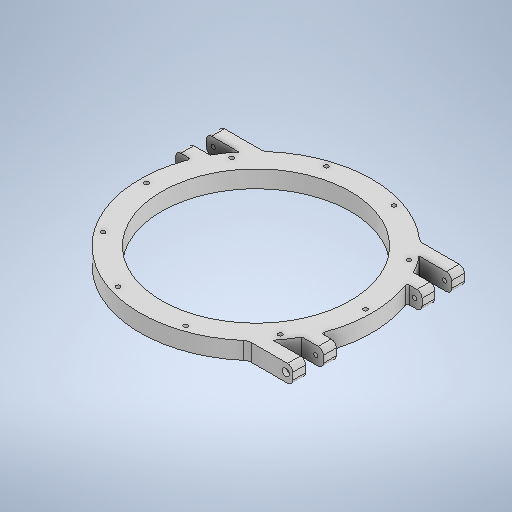
# Autodesk Inventor part: Cylinder 80-20 Spacer_2
Saved by Autodesk Inventor 2025 (Build 290162000, 162)
## iProperties
Created: 2024-04-28
Part Number: Cylinder 80-20 Spacer_2
Material: Generic
Document SubType Name: Modeling
Designer: Thienan Hoang
Density: 1 g/cm^3
Appearance: Default
Author: Thienan Hoang
Autodesk Inventor part; units mm, degrees
ref_plane "YZ Plane" through (0, 0, 0) normal (1, 0, 0) x (0, 1, 0)
ref_plane "XZ Plane" through (0, 0, 0) normal (0, 1, 0) x (-1, 0, 0)
ref_plane "XY Plane" through (0, 0, 0) normal (0, 0, 1) x (1, 0, 0)
sketch "Sketch1" plane through (0, 0, 0) normal (0, 1, 0) x (-1, 0, 0)
  circle A0 centre (0, 0) radius 135
  circle A1 centre (0, 0) radius 110
  dimension "d0" = 270
  dimension "d1" = 220
  constraints: 2 centre point, 2 coincident
  measures "d0" diameter of A0
  measures "d1" diameter of A1
extrude "Extrusion1" add sketch "Sketch1" along normal mid plane 20
sketch "Sketch3" plane through (0, 10, 0) normal (0, 1, 0) x (1, 0, 0)
  circle A0 centre (0, 0) radius 127.5
  circle A1 centre (127.5, 0) radius 2.5
  circle A2 centre (103.1497, 74.9426) radius 2.5
  circle A3 centre (39.3997, 121.2597) radius 2.5
  circle A4 centre (-39.3997, 121.2597) radius 2.5
  circle A5 centre (-103.1497, 74.9426) radius 2.5
  circle A6 centre (-127.5, 0) radius 2.5
  circle A7 centre (-103.1497, -74.9426) radius 2.5
  circle A8 centre (-39.3997, -121.2597) radius 2.5
  circle A9 centre (39.3997, -121.2597) radius 2.5
  circle A10 centre (103.1497, -74.9426) radius 2.5
  dimension "d7" = 255
  dimension "d8" = 5
  dimension "d11" = 360
  constraints: 10 centre point, 1 coincident, 1 horizontal alignment, 23 other
  measures "d8" diameter of A1
hole "Hole1" at (127.5, 10, 0) at (103.1497, 10, 74.9426) at (39.3997, 10, 121.2597) at (-39.3997, 10, 121.2597) at (-103.1497, 10, 74.9426) at (-127.5, 10, 0) at (-103.1497, 10, -74.9426) at (-39.3997, 10, -121.2597) at (39.3997, 10, -121.2597) at (103.1497, 10, -74.9426) direction (0, -1, 0) diameter 5 end through all
sketch "Sketch4" plane through (0, 10, 0) normal (0, 1, 0) x (1, 0, 0)
  circle A0 centre (0, 0) radius 60
  circle A1 centre (103.1497, 74.9426) radius 2.5 projected
  circle A2 centre (39.3997, 121.2597) radius 2.5 projected
  circle A3 centre (-39.3997, 121.2597) radius 2.5 projected
  circle A4 centre (-103.1497, 74.9426) radius 2.5 projected
  circle A5 centre (-127.5, 0) radius 2.5 projected
  circle A6 centre (-103.1497, -74.9426) radius 2.5 projected
  circle A7 centre (-39.3997, -121.2597) radius 2.5 projected
  circle A8 centre (39.3997, -121.2597) radius 2.5 projected
  circle A9 centre (103.1497, -74.9426) radius 2.5 projected
  circle A10 centre (127.5, 0) radius 2.5 projected
  circle A11 centre (0, 0) radius 135 projected
  circle A12 centre (0, 0) radius 110 projected
  line L0 (118.3531, 64.9426) -> (143.3531, 64.9426)
  line L1 (143.3531, 64.9426) -> (143.3531, 49.9426)
  line L2 (143.3531, 49.9426) -> (118.3531, 49.9426)
  line L3 (118.3531, 49.9426) -> (118.3531, 64.9426)
  line L4 (142.6466, 84.9426) -> (90.755, 84.9426)
  line L5 (90.755, 84.9426) -> (90.755, 99.9426)
  line L6 (90.755, 99.9426) -> (142.6466, 99.9426)
  line L7 (142.6466, 99.9426) -> (142.6466, 84.9426)
  line L8 (103.1497, 74.9426) -> (138.3886, 74.9426) construction
  point P0 (125.4222, 49.9426)
  point P1 (104.9274, 84.9426)
  dimension "d21" = 120
  dimension "d22" = 25
  dimension "d23" = 15
  dimension "d24" = 20
  dimension "d25" = 15
  constraints: 18 end point, 4 parallel, 3 horizontal, 2 perpendicular, 2 point on circle, 1 centre point, 1 coincident, 1 other
  measures "d21" diameter of A0
  measures "d22" distance of L1.end L2.end
  measures "d23" distance of L0.end L1.end
  measures "d24" distance between parallel lines of L0 L4
  measures "d25" distance of L6.end L4.start
extrude "Extrusion3" add sketch "Sketch4" against normal up to surface (20 mm away) contours L6 L7 L4 A11 | A11 L0 L1 L2
fillet "Fillet1" radius 6 4 edges at (142.6466, 10, -92.4426) (142.6466, -10, -92.4426) (143.3531, -10, -57.4426) (143.3531, 10, -57.4426)
fillet "Fillet2" radius 10 1 edges at (90.755, 0, -99.9426)
fillet "Fillet3" radius 2 1 edges at (125.4222, 0, -49.9426)
sketch "Sketch5" plane through (142.6466, -4, -99.9426) normal (0, 0, -1) x (-1, 0, 0)
  line L0 (0, 8) -> (0, 0) projected
  line L1 (48.1076, -6) -> (6, -6) projected
  point P0 (142.6466, 4)
  point P1 (8, 4)
  point P2 (0, 4)
  dimension "d38" = 8
  dimension "d39" = 10
  constraints: 1 midpoint
  measures "d38" distance of point (0, 4) point (8, 4)
  measures "d39" distance from line of L1 point (8, 4)
hole "Hole2" at (134.6466, 0, -99.9426) direction (0, 0, 1) diameter 5 depth 50 tip angle 118 counterbore diameter 8.5 counterbore depth 5
mirror "Mirror1" about plane through (0, 0, 0) normal (1, 0, 0) of "Extrusion3", "Fillet1", "Fillet2", "Fillet3", "Hole2"
mirror "Mirror2" about plane through (0, 0, 0) normal (0, 0, 1) of "Extrusion3", "Fillet1", "Fillet2", "Fillet3", "Hole2"
body "Solid1"
